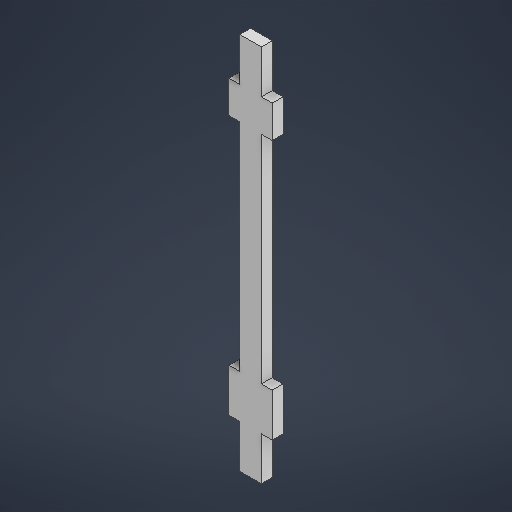
# Autodesk Inventor part: standformiddleslide2
Saved by Autodesk Inventor 2026.2 (Build 302298000, 298)
## iProperties
Created: 2026-04-17
Part Number: standformiddleslide2
Material: Generic
Document SubType Name: Modeling
Designer: danda
Density: 1 g/cm^3
Appearance: Default
Author: danda
Autodesk Inventor part; units mm, degrees
ref_plane "YZ Plane" through (0, 0, 0) normal (1, 0, 0) x (0, 1, 0)
ref_plane "XZ Plane" through (0, 0, 0) normal (0, 1, 0) x (-1, 0, 0)
ref_plane "XY Plane" through (0, 0, 0) normal (0, 0, 1) x (1, 0, 0)
sketch "Sketch1" plane through (0, 0, 0) normal (0, 0, 1) x (1, 0, 0)
  line L0 (-5, 87.5) -> (5, 87.5)
  line L1 (5, 87.5) -> (5, -87.5)
  line L2 (5, -87.5) -> (-5, -87.5)
  line L3 (-5, -87.5) -> (-5, 87.5)
  line L4 (-5, 67.5) -> (-10, 67.5)
  line L5 (-10, 67.5) -> (-10, 52.5)
  line L6 (-10, 52.5) -> (-5, 52.5)
  line L7 (-5, 52.5) -> (-5, 67.5)
  line L8 (5, 67.5) -> (10, 67.5)
  line L9 (10, 67.5) -> (10, 52.5)
  line L10 (10, 52.5) -> (5, 52.5)
  line L11 (5, 52.5) -> (5, 67.5)
  line L12 (-5, -47.5) -> (-10, -47.5)
  line L13 (-10, -47.5) -> (-10, -67.5)
  line L14 (-10, -67.5) -> (-5, -67.5)
  line L15 (-5, -67.5) -> (-5, -47.5)
  line L16 (5, -47.5) -> (10, -47.5)
  line L17 (10, -47.5) -> (10, -67.5)
  line L18 (10, -67.5) -> (5, -67.5)
  line L19 (5, -67.5) -> (5, -47.5)
  point P0 (0, 0)
  point P1 (-7.5, -67.5)
  dimension "d0" = 10
  dimension "d1" = 175
  dimension "d2" = 5
  dimension "d3" = 15
  dimension "d4" = 5
  dimension "d5" = 87.5
  dimension "d6" = 20
  dimension "d7" = 5
  dimension "d8" = 15
  dimension "d9" = 20
  dimension "d10" = 5
  dimension "d11" = 20
  dimension "d12" = 5
  dimension "d13" = 20
  dimension "d14" = 20
  dimension "d16" = 20
  constraints: 40 end point, 10 parallel, 5 horizontal, 5 perpendicular, 4 point on line, 1 midpoint
  measures "d0" distance of L1.end L2.end
  measures "d1" distance of L0.end L1.end
  measures "d2" distance of L6.end L5.end
  measures "d3" distance of L5.end L4.end
  measures "d4" horizontal distance of L1.end point (0, 0)
  measures "d5" vertical distance of L1.end point (0, 0)
  measures "d6" distance between parallel lines of L0 L4
  measures "d7" distance of L9.end L10.end
  measures "d8" distance of L8.end L9.end
  measures "d9" distance from line of L0.end L8
  measures "d10" distance of L14.end L13.end
  measures "d11" distance of L13.end L12.end
  measures "d12" distance of L17.end L18.end
  measures "d13" distance of L16.end L17.end
  measures "d14" distance between parallel lines of L18 L2
  measures "d16" distance from line of L2 point (-7.5, -67.5)
extrude "Extrusion1" add sketch "Sketch1" along normal blind 5
body "Solid1"
